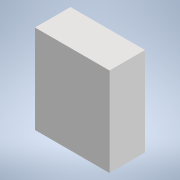
# Autodesk Inventor part: motormount
Saved by Autodesk Inventor 2020 (Build 240168000, 168)
## iProperties
Created: 2022-12-14
Part Number: motormount
Material: Generic
Document SubType Name: Modeling
Designer: Manish
Density: 1 g/cm^3
Appearance: Default
Author: Manish
Autodesk Inventor part; units mm, degrees
ref_plane "YZ Plane" through (0, 0, 0) normal (1, 0, 0) x (0, 1, 0)
ref_plane "XZ Plane" through (0, 0, 0) normal (0, 1, 0) x (-1, 0, 0)
ref_plane "XY Plane" through (0, 0, 0) normal (0, 0, 1) x (1, 0, 0)
sketch "Sketch1" plane through (0, 0, 0) normal (0, 0, 1) x (1, 0, 0)
  line L0 (0, 0) -> (0, -50)
  line L1 (0, -50) -> (82, -50)
  line L2 (82, -50) -> (82, 0)
  line L3 (82, 0) -> (0, 0)
  dimension "d0" = 50
  dimension "d1" = 82
  constraints: 8 end point, 2 parallel, 1 perpendicular, 1 vertical
  measures "d0" distance of L0.start L0.end
  measures "d1" distance of L1.end L0.end
extrude "Extrusion1" add sketch "Sketch1" along normal blind 20
body "Solid1"
